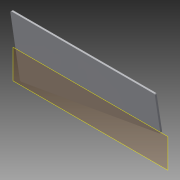
# Autodesk Inventor part: Panel_side
Saved by Autodesk Inventor 2013 (Build 170138000, 138)
## iProperties
Created: 2013-01-31
Part Number: Panel_side
Material: Aluminum 6061
Document SubType Name: Modeling
Designer: xylzlyx
Density: 1 g/cm^3
Author: xylzlyx
Autodesk Inventor part; units mm, degrees
ref_plane "YZ Plane" through (0, 0, 0) normal (1, 0, 0) x (0, 1, 0)
ref_plane "XZ Plane" through (0, 0, 0) normal (0, 1, 0) x (-1, 0, 0)
ref_plane "XY Plane" through (0, 0, 0) normal (0, 0, 1) x (1, 0, 0)
ref_plane "OriginPanel" through (0, 0, 0) normal (0, 0, 1) x (1, 0, 0)
sketch "Sketch1" plane through (0, 0, 0) normal (0, 0, 1) x (1, 0, 0)
  line L0 (-11.9302, 53.3168) -> (-257.9302, 53.3168) projected
  line L1 (-1.9696, -0.3473) -> (-241.005, -42.4957) projected
  line L2 (-257.9302, 53.3168) -> (-241.005, -42.4957)
  line L3 (-1.9696, -0.3473) -> (-11.9302, 53.3168)
  line L4 (-11.9302, 53.3168) -> (-257.9302, 53.3168)
  line L5 (-241.005, -42.4957) -> (-1.9696, -0.3473)
  point P0 (0, 0)
  constraints: 8 end point, 1 collinear
extrude "PanelExtrusion" add sketch "Sketch1" against normal blind 3
fillet "CornerFillet" radius 2 4 edges at (-257.9302, 53.3168, -1.5) (-11.9302, 53.3168, -1.5) (-1.9696, -0.3473, -1.5) (-241.005, -42.4957, -1.5)
body "Solid1"
